# Autodesk Inventor part: rack_test
Saved by Autodesk Inventor 2014 (Build 180170000, 170)
## iProperties
Created: 2015-05-20
Part Number: rack_test
Material: Generic
Document SubType Name: Modeling
Designer: Martin
Density: 1 g/cm^3
Appearance: Default
Author: Martin
Autodesk Inventor part; units mm, degrees
ref_plane "YZ Plane" through (0, 0, 0) normal (1, 0, 0) x (0, 1, 0)
ref_plane "XZ Plane" through (0, 0, 0) normal (0, 1, 0) x (-1, 0, 0)
ref_plane "XY Plane" through (0, 0, 0) normal (0, 0, 1) x (1, 0, 0)
sketch "Sketch1" plane through (0, 0, 0) normal (0, 0, 1) x (1, 0, 0)
  line L0 (0, -9.4281) -> (0, 9.3187)
  arc A0 (6.7496, 0.073) -> (6.51, 0.4187) centre (6.3746, 0.0689) ccw projected
  arc A1 (-6.7496, 0.073) -> (6.7496, 0.073) centre (0, 0) ccw projected
  arc A2 (-6.51, 0.4187) -> (-6.7496, 0.073) centre (-6.3746, 0.0689) ccw projected
  arc A3 (-4.3687, 0.6769) -> (-6.51, 0.4187) centre (-4.9321, -3.658) ccw projected
  arc A4 (-4.3687, 0.6769) -> (-4.2435, 0.7684) centre (-4.3542, 0.7885) ccw projected
  arc A5 (-4.2145, 0.914) -> (-4.2435, 0.7684) centre (0, 0) ccw projected
  arc A6 (-4.2145, 0.914) -> (-4.2952, 1.0464) centre (-4.3245, 0.9378) ccw projected
  arc A7 (-6.1747, 2.1045) -> (-4.2952, 1.0464) centre (-3.1568, 5.267) ccw projected
  arc A8 (-6.2638, 2.5155) -> (-6.1747, 2.1045) centre (-5.9158, 2.3758) ccw projected
  arc A9 (-6.0212, 3.0507) -> (-6.2638, 2.5155) centre (0, 0) ccw projected
  arc A10 (-5.6535, 3.2548) -> (-6.0212, 3.0507) centre (-5.6867, 2.8813) ccw projected
  arc A11 (-3.6188, 2.5393) -> (-5.6535, 3.2548) centre (-6.0413, -1.0993) ccw projected
  arc A12 (-3.6188, 2.5393) -> (-3.466, 2.566) centre (-3.5564, 2.633) ccw projected
  arc A13 (-3.3757, 2.6838) -> (-3.466, 2.566) centre (0, 0) ccw projected
  arc A14 (-3.3757, 2.6838) -> (-3.3894, 2.8382) centre (-3.4637, 2.7538) ccw projected
  arc A15 (-4.6071, 4.6184) -> (-3.3894, 2.8382) centre (-0.5017, 6.12) ccw projected
  arc A16 (-4.5052, 5.0265) -> (-4.6071, 4.6184) centre (-4.2549, 4.7472) ccw projected
  arc A17 (-4.051, 5.3993) -> (-4.5052, 5.0265) centre (0, 0) ccw projected
  arc A18 (-3.6309, 5.4196) -> (-4.051, 5.3993) centre (-3.8259, 5.0993) ccw projected
  arc A19 (-2.1225, 3.878) -> (-3.6309, 5.4196) centre (-5.9045, 1.6861) ccw projected
  arc A20 (-2.1225, 3.878) -> (-1.9736, 3.8344) centre (-2.0251, 3.9344) ccw projected
  arc A21 (-1.8405, 3.9) -> (-1.9736, 3.8344) centre (0, 0) ccw projected
  arc A22 (-1.8405, 3.9) -> (-1.7845, 4.0446) centre (-1.8886, 4.0017) ccw projected
  arc A23 (-2.0893, 6.1798) -> (-1.7845, 4.0446) centre (2.2568, 5.7108) ccw projected
  arc A24 (-1.8174, 6.5007) -> (-2.0893, 6.1798) centre (-1.7165, 6.1396) ccw projected
  arc A25 (-1.2452, 6.6342) -> (-1.8174, 6.5007) centre (0, 0) ccw projected
  arc A26 (-0.8594, 6.4666) -> (-1.2452, 6.6342) centre (-1.176, 6.2656) ccw projected
  arc A27 (-0.1884, 4.4168) -> (-0.8594, 6.4666) centre (-4.5499, 4.1237) ccw projected
  arc A28 (-0.1884, 4.4168) -> (-0.0742, 4.3119) centre (-0.0761, 4.4243) ccw projected
  arc A29 (0.0742, 4.3119) -> (-0.0742, 4.3119) centre (0, 0) ccw projected
  arc A30 (0.0742, 4.3119) -> (0.1884, 4.4168) centre (0.0761, 4.4243) ccw projected
  arc A31 (0.8594, 6.4666) -> (0.1884, 4.4168) centre (4.5499, 4.1237) ccw projected
  arc A32 (1.2452, 6.6342) -> (0.8594, 6.4666) centre (1.176, 6.2656) ccw projected
  arc A33 (1.8174, 6.5007) -> (1.2452, 6.6342) centre (0, 0) ccw projected
  arc A34 (2.0893, 6.1798) -> (1.8174, 6.5007) centre (1.7165, 6.1396) ccw projected
  arc A35 (1.7845, 4.0446) -> (2.0893, 6.1798) centre (-2.2568, 5.7108) ccw projected
  arc A36 (1.7845, 4.0446) -> (1.8405, 3.9) centre (1.8886, 4.0017) ccw projected
  arc A37 (1.9736, 3.8344) -> (1.8405, 3.9) centre (0, 0) ccw projected
  arc A38 (1.9736, 3.8344) -> (2.1225, 3.878) centre (2.0251, 3.9344) ccw projected
  arc A39 (3.6309, 5.4196) -> (2.1225, 3.878) centre (5.9045, 1.6861) ccw projected
  arc A40 (4.051, 5.3993) -> (3.6309, 5.4196) centre (3.8259, 5.0993) ccw projected
  arc A41 (4.5052, 5.0265) -> (4.051, 5.3993) centre (0, 0) ccw projected
  arc A42 (4.6071, 4.6184) -> (4.5052, 5.0265) centre (4.2549, 4.7472) ccw projected
  arc A43 (3.3894, 2.8382) -> (4.6071, 4.6184) centre (0.5017, 6.12) ccw projected
  arc A44 (3.3894, 2.8382) -> (3.3757, 2.6838) centre (3.4637, 2.7538) ccw projected
  arc A45 (3.466, 2.566) -> (3.3757, 2.6838) centre (0, 0) ccw projected
  arc A46 (3.466, 2.566) -> (3.6188, 2.5393) centre (3.5564, 2.633) ccw projected
  arc A47 (5.6535, 3.2548) -> (3.6188, 2.5393) centre (6.0413, -1.0993) ccw projected
  arc A48 (6.0212, 3.0507) -> (5.6535, 3.2548) centre (5.6867, 2.8813) ccw projected
  arc A49 (6.2638, 2.5155) -> (6.0212, 3.0507) centre (0, 0) ccw projected
  arc A50 (6.1747, 2.1045) -> (6.2638, 2.5155) centre (5.9158, 2.3758) ccw projected
  arc A51 (4.2952, 1.0464) -> (6.1747, 2.1045) centre (3.1568, 5.267) ccw projected
  arc A52 (4.2952, 1.0464) -> (4.2145, 0.914) centre (4.3245, 0.9378) ccw projected
  arc A53 (4.2435, 0.7684) -> (4.2145, 0.914) centre (0, 0) ccw projected
  arc A54 (4.2435, 0.7684) -> (4.3687, 0.6769) centre (4.3542, 0.7885) ccw projected
  arc A55 (6.51, 0.4187) -> (4.3687, 0.6769) centre (4.9321, -3.658) ccw projected
  circle A56 centre (0, 0) radius 1.5 projected
  line L1 (-10, 6.8906) -> (10, 6.8906)
  line L2 (-10, 6.8906) -> (-10, 7.8906)
  line L3 (-10, 7.8906) -> (10, 7.8906)
  line L4 (10, 7.8906) -> (10, 6.8906)
  line L5 (-10, 6.6406) -> (10, 6.6406) construction
  line L6 (0, 4.7099) -> (-1.3614, 7.6295) construction
  line L7 (-0.5881, 5.9711) -> (0.5881, 5.9711) construction
  line L8 (-1.4832, 7.8906) -> (0, 4.7099) construction
  line L9 (0.5881, 5.9711) -> (-0.5881, 5.9711) construction
  arc A57 (-0.7, 6.8906) -> (-0.1371, 5.2406) centre (7.2211, 8.6718) ccw
  line L10 (-0.1371, 5.2406) -> (0.1371, 5.2406)
  arc A58 (0.1371, 5.2406) -> (0.7, 6.8906) centre (-7.2211, 8.6718) ccw
  line L11 (-1.3728, 7.8906) -> (0, 4.9465) construction
  point P0 (0, 6.8906)
  dimension "d0" = 20
  dimension "d1" = 0.25
  dimension "d2" = 1
  dimension "d3" = 0.1
  dimension "d4" = 1.4
  dimension "d5" = 1.65
  constraints: 20 end point, 7 point on line, 5 perpendicular, 4 point on circle, 2 centre point, 2 collinear, 2 parallel, 2 tangent, 1 midpoint, 1 symmetric about line, 1 vertical, 3 other
  measures "d0" distance of L1.start L1.end
  measures "d1" distance between parallel lines of L5 L1
  measures "d2" distance between parallel lines of L1 L3
  measures "d3" distance between parallel lines of L8 L11
  measures "d4" distance of A58.end A57.start
  measures "d5" distance between parallel lines of L1 L10
extrude "Extrusion1" add sketch "Sketch1" along normal blind 6 contours L10 A57 L1 L0 | L0 L1 A58 L10
sketch "Sketch3" plane through (0, 0, 0) normal (0, 0, 1) x (1, 0, 0)
  line L0 (-10, 7.8906) -> (10, 7.8906) projected
  line L1 (-10, 6.8906) -> (-10, 7.8906) projected
  line L2 (-10, 6.8906) -> (10, 6.8906) projected
  line L3 (10, 7.8906) -> (10, 6.8906) projected
  point P0 (0, 0)
extrude "Extrusion2" add sketch "Sketch3" along normal up to surface (6 mm away)
pattern_linear "Rectangular Pattern1" count 7 spacing 2.7 along (1, 0, 0) of "Extrusion1" first direction both ways yes
equation "\"d12\" = 3.6 * model_gear_module"
equation "\"model_gear_module\" = 0.75"
body "Solid1"
